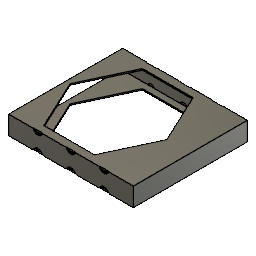
NES Shelf v3 (Autodesk Fusion 360 design; units mm, degrees)
Autodesk Fusion 360 part; units mm, degrees
(part 1 of 2)
sketch "Sketch1" plane through (0, 0, 0) normal (0, 1, 0) x (1, 0, 0)
  line L0 (0, 0) -> (133.9, 0)
  line L1 (133.9, 0) -> (133.9, -119.82)
  line L2 (133.9, -119.82) -> (0, -119.82)
  line L3 (0, -119.82) -> (0, 0)
  line L4 (0, -59.91) -> (109.9, -59.91)
  line L5 (109.9, -59.91) -> (109.9, -6.71)
  line L6 (109.9, -6.71) -> (0, -6.71)
  line L7 (0, -6.71) -> (0, -59.91)
  line L8 (0, -59.91) -> (109.9, -59.91)
  line L9 (109.9, -59.91) -> (109.9, -113.11)
  line L10 (109.9, -113.11) -> (0, -113.11)
  line L11 (0, -113.11) -> (0, -59.91)
  line L12 (109.9, -6.71) -> (109.9, 0)
  line L13 (109.9, -113.11) -> (109.9, -119.82)
  line L14 (109.9, -119.82) -> (109.9, -113.11)
  line L15 (133.9, -113.11) -> (109.9, -113.11)
  line L16 (109.9, -6.71) -> (133.9, -6.71)
  dimension "d1" = 119.82
  dimension "d2" = 133.9
  dimension "d3" = 53.2
  dimension "d4" = 109.9
  dimension "d5" = 53.2
  constraint horizontal L0
  constraint vertical L1
  constraint horizontal L2
  constraint vertical L3
  constraint coincident L0.start L3.end
  constraint horizontal L4
  constraint vertical L5
  constraint horizontal L6
  constraint vertical L7
  constraint midpoint L3 L4.start
  constraint horizontal L8
  constraint vertical L9
  constraint horizontal L10
  constraint vertical L11
  constraint coincident L0 L12.end
  constraint perpendicular L0 L12
  constraint coincident L2 L13.end
  constraint perpendicular L2 L13
  constraint coincident L1 L15.start
  constraint perpendicular L9 L15
  constraint coincident L1 L16.end
  constraint perpendicular L1 L16
  measures "d1" distance of L0.start L2.end
  measures "d2" distance of L0.start L0.end
  measures "d3" distance of L4.start L6.end
  measures "d4" distance of L4.start L4.end
  measures "d5" distance of L4.start L10.end
extrude "Extrude1" add sketch "Sketch1" along normal blind 16.8 contours L0 L3 L6 L12 | L3 L4 L5 L6 L7 L8 | L1 L5 L9 L15 L16 | L3 L4 L8 L9 L10 L11 | L2 L3 L10 L13 L14 makes body 1
sketch "Sketch2" plane through (0, 0, 0) normal (0, 1, 0) x (1, 0, 0)
  line L0 (0, 0) -> (133.9, 0)
  line L1 (133.9, 0) -> (133.9, -119.82)
  line L2 (133.9, -119.82) -> (0, -119.82)
  line L3 (0, -119.82) -> (0, 0)
  line L4 (133.9, 0) -> (135.9, 0)
  line L5 (135.9, 0) -> (135.9, -119.82)
  line L6 (135.9, -119.82) -> (133.9, -119.82)
  line L7 (133.9, -119.82) -> (133.9, 0)
  line L8 (135.9, 0) -> (0, 0)
  line L9 (0, 0) -> (0, 2)
  line L10 (0, 2) -> (135.9, 2)
  line L11 (135.9, 2) -> (135.9, 0)
  line L12 (135.9, -119.82) -> (0, -119.82)
  line L13 (0, -119.82) -> (0, -121.82)
  line L14 (0, -121.82) -> (135.9, -121.82)
  line L15 (135.9, -121.82) -> (135.9, -119.82)
  line L16 (133.9, 0) -> (110.1, 0)
  line L17 (110.1, 0) -> (110.1, -6.5)
  line L18 (110.1, -6.5) -> (133.9, -6.5)
  line L19 (133.9, -6.5) -> (133.9, 0)
  line L20 (133.9, -119.82) -> (110.1, -119.82)
  line L21 (110.1, -119.82) -> (110.1, -113.32)
  line L22 (110.1, -113.32) -> (133.9, -113.32)
  line L23 (133.9, -113.32) -> (133.9, -119.82)
  dimension "d8" = 133.9
  dimension "d9" = 2
  dimension "d10" = 2
  dimension "d11" = 2
  dimension "d12" = 23.8
  dimension "d13" = 6.5
  dimension "d14" = 23.8
  dimension "d15" = 6.5
  constraint horizontal L0
  constraint vertical L1
  constraint horizontal L2
  constraint vertical L3
  constraint coincident L0.start L3.end
  constraint horizontal L4
  constraint vertical L5
  constraint horizontal L6
  constraint vertical L7
  constraint horizontal L8
  constraint vertical L9
  constraint horizontal L10
  constraint vertical L11
  constraint horizontal L12
  constraint vertical L13
  constraint horizontal L14
  constraint vertical L15
  constraint horizontal L16
  constraint vertical L17
  constraint horizontal L18
  constraint vertical L19
  constraint horizontal L20
  constraint vertical L21
  constraint horizontal L22
  constraint vertical L23
  measures "d8" distance of L0.start L0.end
  measures "d9" distance of L0.end L4.end
  measures "d10" distance of L4.end L10.end
  measures "d11" distance of L5.end L14.end
  measures "d12" distance of L0.end L16.end
  measures "d13" distance of L0.end L18.end
  measures "d14" distance of L1.end L20.end
  measures "d15" distance of L1.end L22.end
extrude "Extrude2" add sketch "Sketch2" along normal blind 17 separate body contours L0 L4 L8 L9 L10 L11 L16 | L0 L1 L7 L8 L16 L17 L18 L19 | L2 L6 L12 L13 L14 L15 L20 | L1 L4 L5 L6 L7 L8 L12 L19 L23 | L1 L2 L7 L12 L20 L21 L22 L23 makes body 2
extrude "Extrude3" cut 1 faces at (36.7, 11.3333, 0) along direction (0, 0, -1) blind 0.2 on bodies 2 bodies 2
extrude "Extrude4" cut 1 faces at (73.4, 5.6667, 119.82) along direction (0, 0, 1) blind 0.2 on bodies 2 bodies 2
extrude "Extrude5" add 1 faces at (45.3, 5.6667, -2) along direction (0, 0, -1) blind 0.2 on bodies 2 bodies 2
extrude "Extrude6" add 1 faces at (45.3, 5.6667, 121.82) along direction (0, 0, 1) blind 0.2 on bodies 2 bodies 2
sketch "Sketch3" plane through (0, 0, 0) normal (0, -1, 0) x (1, 0, 0)
  line L0 (110.1, 120.02) -> (110.1, 113.32)
  line L1 (110.1, 113.32) -> (133.9, 113.32)
  line L2 (133.9, 113.32) -> (133.9, 6.5)
  line L3 (133.9, 6.5) -> (110.1, 6.5)
  line L4 (110.1, 6.5) -> (110.1, -0.2)
  line L5 (110.1, -0.2) -> (0, -0.2)
  line L6 (0, -0.2) -> (0, -2.2)
  line L7 (0, -2.2) -> (135.9, -2.2)
  line L8 (135.9, -2.2) -> (135.9, 122.02)
  line L9 (135.9, 122.02) -> (0, 122.02)
  line L10 (0, 122.02) -> (0, 120.02)
  line L11 (0, 120.02) -> (110.1, 120.02)
  line L12 (135.9, -2.2) -> (0, -2.2)
  line L13 (0, -2.2) -> (0, 122.02)
  line L14 (0, 122.02) -> (135.9, 122.02)
  line L15 (135.9, 122.02) -> (135.9, -2.2)
  constraint horizontal L12
  constraint vertical L13
  constraint horizontal L14
  constraint vertical L15
  constraint coincident L9.end L10.start
  constraint coincident L7.end L8.start
extrude "Extrude7" add sketch "Sketch3" along normal blind 1.5 bodies 2
sketch "Sketch4" plane through (0, 17, 0) normal (0, 1, 0) x (-1, 0, 0)
  line L0 (-110.1, 113.32) -> (-110.1, 120.02)
  line L1 (-110.1, 120.02) -> (0, 120.02)
  line L2 (0, 120.02) -> (0, 122.02)
  line L3 (0, 122.02) -> (-135.9, 122.02)
  line L4 (-135.9, 122.02) -> (-135.9, -2.2)
  line L5 (-135.9, -2.2) -> (0, -2.2)
  line L6 (0, -2.2) -> (0, -0.2)
  line L7 (0, -0.2) -> (-110.1, -0.2)
  line L8 (-110.1, -0.2) -> (-110.1, 6.5)
  line L9 (-110.1, 6.5) -> (-133.9, 6.5)
  line L10 (-133.9, 6.5) -> (-133.9, 113.32)
  line L11 (-133.9, 113.32) -> (-110.1, 113.32)
  line L12 (-135.9, -2.2) -> (0, -2.2)
  line L13 (0, -2.2) -> (0, 122.02)
  line L14 (0, 122.02) -> (-135.9, 122.02)
  line L15 (-135.9, 122.02) -> (-135.9, -2.2)
  constraint horizontal L12
  constraint vertical L13
  constraint horizontal L14
  constraint vertical L15
  constraint coincident L2.end L3.start
  constraint coincident L4.end L5.start
extrude "Extrude8" add sketch "Sketch4" along normal blind 1.5 bodies 2
extrude "Extrude9" cut 1 faces at (45.3, 18.5, 39.2067) along direction (0, -1, 0) blind 0.5 on bodies 2 bodies 2
extrude "Extrude10" cut 1 faces at (90.6, -1.5, 39.2067) along direction (0, 1, 0) blind 0.5 on bodies 2 bodies 2
sketch "Sketch5" plane through (0, 0, -2.2) normal (0, 0, -1) x (-1, 0, 0)
  line L0 (-135.9, -1) -> (0, -1)
  line L1 (0, -1) -> (0, 18)
  line L2 (0, 18) -> (-135.9, 18)
  line L3 (-135.9, 18) -> (-135.9, -1)
  line L4 (-67.95, -1) -> (-63.95, -1)
  line L5 (-63.95, -1) -> (-63.95, 0)
  line L6 (-63.95, 0) -> (-67.95, 0)
  line L7 (-67.95, 0) -> (-67.95, -1)
  line L8 (-67.95, 0) -> (-71.95, 0)
  line L9 (-71.95, 0) -> (-71.95, -1)
  line L10 (-71.95, -1) -> (-67.95, -1)
  line L11 (-67.95, -1) -> (-67.95, 0)
  line L12 (-63.95, 0) -> (-71.95, 0)
  line L13 (-71.95, 0) -> (-71.95, 2)
  line L14 (-71.95, 2) -> (-63.95, 2)
  line L15 (-63.95, 2) -> (-63.95, 0)
  dimension "d34" = 4
  dimension "d35" = 1
  dimension "d36" = 1
  dimension "d37" = 4
  dimension "d38" = 8
  dimension "d39" = 2
  constraint horizontal L4
  constraint vertical L5
  constraint horizontal L6
  constraint vertical L7
  constraint midpoint L0 L4.start
  constraint horizontal L8
  constraint vertical L9
  constraint horizontal L10
  constraint vertical L11
  constraint horizontal L12
  constraint vertical L13
  constraint horizontal L14
  constraint vertical L15
  measures "d34" distance of L4.start L4.end
  measures "d35" distance of L4.start L6.end
  measures "d36" distance of L6.end L4.start
  measures "d37" distance of L6.end L8.end
  measures "d38" distance of L5.end L8.end
  measures "d39" distance of L5.end L14.end
extrude "Extrude11" cut sketch "Sketch5" against normal blind 1.5 contours L6 L8 L12 L13 L14 L15 bodies 2
extrude "Extrude12" cut sketch "Sketch5" against normal blind 0.5 contours L0 L7 L8 L9 L10 L11 L12 | L0 L4 L5 L6 L7 L11 L12 bodies 2
sketch "Sketch6" plane through (0, 0, -2.2) normal (0, 0, -1) x (-1, 0, 0)
  line L0 (-71.95, -1) -> (-71.95, 2)
  line L1 (-71.95, 2) -> (-63.95, 2)
  line L2 (-63.95, 2) -> (-63.95, -1)
  line L3 (-63.95, -1) -> (0, -1)
  line L4 (0, -1) -> (0, 18)
  line L5 (0, 18) -> (-135.9, 18)
  line L6 (-135.9, 18) -> (-135.9, -1)
  line L7 (-135.9, -1) -> (-71.95, -1)
  line L8 (-31.975, -1) -> (-27.975, -1)
  line L9 (-27.975, -1) -> (-27.975, 0)
  line L10 (-27.975, 0) -> (-31.975, 0)
  line L11 (-31.975, 0) -> (-31.975, -1)
  line L12 (-31.975, 0) -> (-35.975, 0)
  line L13 (-35.975, 0) -> (-35.975, -1)
  line L14 (-35.975, -1) -> (-31.975, -1)
  line L15 (-31.975, -1) -> (-31.975, 0)
  line L16 (-103.925, -1) -> (-99.925, -1)
  line L17 (-99.925, -1) -> (-99.925, 0)
  line L18 (-99.925, 0) -> (-103.925, 0)
  line L19 (-103.925, 0) -> (-103.925, -1)
  line L20 (-103.925, 0) -> (-107.925, 0)
  line L21 (-107.925, 0) -> (-107.925, -1)
  line L22 (-107.925, -1) -> (-103.925, -1)
  line L23 (-103.925, -1) -> (-103.925, 0)
  line L24 (-107.925, 0) -> (-103.925, 0)
  line L25 (-103.925, 0) -> (-103.925, 2)
  line L26 (-103.925, 2) -> (-107.925, 2)
  line L27 (-107.925, 2) -> (-107.925, 0)
  line L28 (-27.975, 0) -> (-35.975, 0)
  line L29 (-35.975, 0) -> (-35.975, 2)
  line L30 (-35.975, 2) -> (-27.975, 2)
  line L31 (-27.975, 2) -> (-27.975, 0)
  line L32 (-103.925, 2) -> (-99.925, 2)
  line L33 (-99.925, 2) -> (-99.925, 0)
  line L34 (-99.925, 0) -> (-103.925, 0)
  line L35 (-103.925, 0) -> (-103.925, 2)
  dimension "d44" = 4
  dimension "d45" = 1
  dimension "d46" = 4
  dimension "d47" = 4
  dimension "d48" = 4
  dimension "d49" = 4
  dimension "d50" = 8
  constraint horizontal L8
  constraint vertical L9
  constraint horizontal L10
  constraint vertical L11
  constraint midpoint L3 L8.start
  constraint horizontal L12
  constraint vertical L13
  constraint horizontal L14
  constraint vertical L15
  constraint horizontal L16
  constraint vertical L17
  constraint horizontal L18
  constraint vertical L19
  constraint midpoint L7 L16.start
  constraint horizontal L20
  constraint vertical L21
  constraint horizontal L22
  constraint vertical L23
  constraint horizontal L24
  constraint vertical L25
  constraint horizontal L26
  constraint vertical L27
  constraint horizontal L28
  constraint vertical L29
  constraint horizontal L30
  constraint vertical L31
  constraint horizontal L32
  constraint vertical L33
  constraint horizontal L34
  constraint vertical L35
  measures "d44" distance of L8.start L8.end
  measures "d45" distance of L8.start L10.end
  measures "d46" distance of L10.end L12.end
  measures "d47" distance of L16.start L16.end
  measures "d48" distance of L18.end L20.end
  measures "d49" distance of L20.end L18.end
  measures "d50" distance of L9.end L12.end
extrude "Extrude13" cut sketch "Sketch6" against normal blind 1.5 contours L18 L25 L32 L33 L34 L35 | L20 L24 L25 L26 L27 L35 | L10 L12 L28 L29 L30 L31 bodies 2
extrude "Extrude14" cut sketch "Sketch6" against normal blind 0.5 contours L7 L16 L17 L18 L19 L23 L34 | L7 L19 L20 L21 L22 L23 L24 | L3 L11 L12 L13 L14 L15 L28 | L3 L8 L9 L10 L11 L15 L28 bodies 2
sketch "Sketch7" plane through (135.9, 0, 0) normal (1, 0, 0) x (0, 0, -1)
  line L0 (-122.02, -1) -> (2.2, -1)
  line L1 (2.2, -1) -> (2.2, 18)
  line L2 (2.2, 18) -> (-122.02, 18)
  line L3 (-122.02, 18) -> (-122.02, -1)
  line L4 (-59.91, -1) -> (-55.91, -1)
  line L5 (-55.91, -1) -> (-55.91, 0)
  line L6 (-55.91, 0) -> (-59.91, 0)
  line L7 (-59.91, 0) -> (-59.91, -1)
  line L8 (-59.91, 0) -> (-63.91, 0)
  line L9 (-63.91, 0) -> (-63.91, -1)
  line L10 (-63.91, -1) -> (-59.91, -1)
  line L11 (-59.91, -1) -> (-59.91, 0)
  line L12 (-63.91, 0) -> (-55.91, 0)
  line L13 (-55.91, 0) -> (-55.91, 2)
  line L14 (-55.91, 2) -> (-63.91, 2)
  line L15 (-63.91, 2) -> (-63.91, 0)
  dimension "d55" = 4
  dimension "d56" = 4
  dimension "d57" = 1
  dimension "d58" = 8
  dimension "d59" = 2
  constraint horizontal L4
  constraint vertical L5
  constraint horizontal L6
  constraint vertical L7
  constraint midpoint L0 L4.start
  constraint horizontal L8
  constraint vertical L9
  constraint horizontal L10
  constraint vertical L11
  constraint horizontal L12
  constraint vertical L13
  constraint horizontal L14
  constraint vertical L15
  measures "d55" distance of L4.start L4.end
  measures "d56" distance of L6.end L8.end
  measures "d57" distance of L6.end L4.start
  measures "d58" distance of L8.end L5.end
  measures "d59" distance of L8.end L14.end
extrude "Extrude15" cut sketch "Sketch7" against normal blind 1.5 contours L6 L8 L12 L13 L14 L15 bodies 2
extrude "Extrude16" cut sketch "Sketch7" against normal blind 0.5 contours L0 L7 L8 L9 L10 L11 L12 | L0 L4 L5 L6 L7 L11 L12 bodies 2
sketch "Sketch8" plane through (135.9, 0, 0) normal (1, 0, 0) x (0, 0, -1)
  line L0 (-55.91, 2) -> (-55.91, -1)
  line L1 (-55.91, -1) -> (2.2, -1)
  line L2 (2.2, -1) -> (2.2, 18)
  line L3 (2.2, 18) -> (-122.02, 18)
  line L4 (-122.02, 18) -> (-122.02, -1)
  line L5 (-122.02, -1) -> (-63.91, -1)
  line L6 (-63.91, -1) -> (-63.91, 2)
  line L7 (-63.91, 2) -> (-55.91, 2)
  line L8 (-26.855, -1) -> (-22.855, -1)
  line L9 (-22.855, -1) -> (-22.855, 0)
  line L10 (-22.855, 0) -> (-26.855, 0)
  line L11 (-26.855, 0) -> (-26.855, -1)
  line L12 (-26.855, 0) -> (-30.855, 0)
  line L13 (-30.855, 0) -> (-30.855, -1)
  line L14 (-30.855, -1) -> (-26.855, -1)
  line L15 (-26.855, -1) -> (-26.855, 0)
  line L16 (-30.855, 0) -> (-22.855, 0)
  line L17 (-22.855, 0) -> (-22.855, 2)
  line L18 (-22.855, 2) -> (-30.855, 2)
  line L19 (-30.855, 2) -> (-30.855, 0)
  line L20 (-92.965, -1) -> (-96.965, -1)
  line L21 (-96.965, -1) -> (-96.965, 0)
  line L22 (-96.965, 0) -> (-92.965, 0)
  line L23 (-92.965, 0) -> (-92.965, -1)
  line L24 (-92.965, 0) -> (-88.965, 0)
  line L25 (-88.965, 0) -> (-88.965, -1)
  line L26 (-88.965, -1) -> (-92.965, -1)
  line L27 (-92.965, -1) -> (-92.965, 0)
  line L28 (-88.965, 0) -> (-96.965, 0)
  line L29 (-96.965, 0) -> (-96.965, 2)
  line L30 (-96.965, 2) -> (-88.965, 2)
  line L31 (-88.965, 2) -> (-88.965, 0)
  dimension "d64" = 4
  dimension "d65" = 4
  dimension "d66" = 8
  dimension "d67" = 2
  dimension "d68" = 4
  dimension "d69" = 4
  dimension "d70" = 1
  dimension "d71" = 8
  dimension "d72" = 2
  constraint horizontal L8
  constraint vertical L9
  constraint horizontal L10
  constraint vertical L11
  constraint midpoint L1 L8.start
  constraint horizontal L12
  constraint vertical L13
  constraint horizontal L14
  constraint vertical L15
  constraint horizontal L16
  constraint vertical L17
  constraint horizontal L18
  constraint vertical L19
  constraint horizontal L20
  constraint vertical L21
  constraint horizontal L22
  constraint vertical L23
  constraint midpoint L5 L20.start
  constraint horizontal L24
  constraint vertical L25
  constraint horizontal L26
  constraint vertical L27
  constraint horizontal L28
  constraint vertical L29
  constraint horizontal L30
  constraint vertical L31
  measures "d64" distance of L8.start L8.end
  measures "d65" distance of L10.end L12.end
  measures "d66" distance of L12.end L9.end
  measures "d67" distance of L12.end L18.end
  measures "d68" distance of L20.start L20.end
  measures "d69" distance of L22.end L24.end
  measures "d70" distance of L22.end L20.start
  measures "d71" distance of L24.end L21.end
  measures "d72" distance of L24.end L30.end
extrude "Extrude17" cut sketch "Sketch8" against normal blind 1.5 contours L10 L12 L16 L17 L18 L19 | L22 L24 L28 L29 L30 L31 bodies 2
extrude "Extrude18" cut sketch "Sketch8" against normal blind 0.5 contours L1 L11 L12 L13 L14 L15 L16 | L1 L8 L9 L10 L11 L15 L16 | L5 L23 L24 L25 L26 L27 L28 | L5 L20 L21 L22 L23 L27 L28 bodies 2
sketch "Sketch9" plane through (0, 0, 122.02) normal (0, 0, 1) x (1, 0, 0)
  line L0 (0, -1) -> (135.9, -1)
  line L1 (135.9, -1) -> (135.9, 18)
  line L2 (135.9, 18) -> (0, 18)
  line L3 (0, 18) -> (0, -1)
  line L4 (67.95, -1) -> (63.95, -1)
  line L5 (63.95, -1) -> (63.95, 0)
  line L6 (63.95, 0) -> (67.95, 0)
  line L7 (67.95, 0) -> (67.95, -1)
  line L8 (67.95, 0) -> (71.95, 0)
  line L9 (71.95, 0) -> (71.95, -1)
  line L10 (71.95, -1) -> (67.95, -1)
  line L11 (67.95, -1) -> (67.95, 0)
  line L12 (71.95, 0) -> (63.95, 0)
  line L13 (63.95, 0) -> (63.95, 2)
  line L14 (63.95, 2) -> (71.95, 2)
  line L15 (71.95, 2) -> (71.95, 0)
  dimension "d77" = 1
  dimension "d78" = 4
  dimension "d79" = 1
  dimension "d80" = 4
  dimension "d81" = 2
  constraint horizontal L4
  constraint vertical L5
  constraint horizontal L6
  constraint vertical L7
  constraint midpoint L0 L4.start
  constraint horizontal L8
  constraint vertical L9
  constraint horizontal L10
  constraint vertical L11
  constraint horizontal L12
  constraint vertical L13
  constraint horizontal L14
  constraint vertical L15
  measures "d77" distance of L4.start L6.end
  measures "d78" distance of L4.start L4.end
  measures "d79" distance of L6.end L4.start
  measures "d80" distance of L6.end L8.end
  measures "d81" distance of L8.end L14.end
extrude "Extrude19" cut sketch "Sketch9" against normal blind 1.5 contours L6 L8 L12 L13 L14 L15 bodies 2
extrude "Extrude20" cut sketch "Sketch9" against normal blind 0.5 contours L0 L4 L5 L6 L7 L11 L12 | L0 L7 L8 L9 L10 L11 L12 bodies 2
sketch "Sketch10" plane through (0, 0, 122.02) normal (0, 0, 1) x (1, 0, 0)
  line L0 (71.95, 2) -> (71.95, -1)
  line L1 (71.95, -1) -> (135.9, -1)
  line L2 (135.9, -1) -> (135.9, 18)
  line L3 (135.9, 18) -> (0, 18)
  line L4 (0, 18) -> (0, -1)
  line L5 (0, -1) -> (63.95, -1)
  line L6 (63.95, -1) -> (63.95, 2)
  line L7 (63.95, 2) -> (71.95, 2)
  line L8 (31.975, -1) -> (35.975, -1)
  line L9 (35.975, -1) -> (35.975, 0)
  line L10 (35.975, 0) -> (31.975, 0)
  line L11 (31.975, 0) -> (31.975, -1)
  line L12 (31.975, 0) -> (27.975, 0)
  line L13 (27.975, 0) -> (27.975, -1)
  line L14 (27.975, -1) -> (31.975, -1)
  line L15 (31.975, -1) -> (31.975, 0)
  line L16 (27.975, 0) -> (35.975, 0)
  line L17 (35.975, 0) -> (35.975, 2)
  line L18 (35.975, 2) -> (27.975, 2)
  line L19 (27.975, 2) -> (27.975, 0)
  line L20 (103.925, -1) -> (107.925, -1)
  line L21 (107.925, -1) -> (107.925, 0)
  line L22 (107.925, 0) -> (103.925, 0)
  line L23 (103.925, 0) -> (103.925, -1)
  line L24 (103.925, 0) -> (99.925, 0)
  line L25 (99.925, 0) -> (99.925, -1)
  line L26 (99.925, -1) -> (103.925, -1)
  line L27 (103.925, -1) -> (103.925, 0)
  line L28 (99.925, 0) -> (107.925, 0)
  line L29 (107.925, 0) -> (107.925, 2)
  line L30 (107.925, 2) -> (99.925, 2)
  line L31 (99.925, 2) -> (99.925, 0)
  dimension "d86" = 4
  dimension "d87" = 4
  dimension "d88" = 1
  dimension "d89" = 8
  dimension "d90" = 2
  dimension "d91" = 4
  dimension "d92" = 4
  dimension "d93" = 8
  constraint horizontal L8
  constraint vertical L9
  constraint horizontal L10
  constraint vertical L11
  constraint midpoint L5 L8.start
  constraint horizontal L12
  constraint vertical L13
  constraint horizontal L14
  constraint vertical L15
  constraint horizontal L16
  constraint vertical L17
  constraint horizontal L18
  constraint vertical L19
  constraint horizontal L20
  constraint vertical L21
  constraint horizontal L22
  constraint vertical L23
  constraint midpoint L1 L20.start
  constraint horizontal L24
  constraint vertical L25
  constraint horizontal L26
  constraint vertical L27
  constraint horizontal L28
  constraint vertical L29
  constraint horizontal L30
  constraint vertical L31
  measures "d86" distance of L8.start L8.end
  measures "d87" distance of L10.end L12.end
  measures "d88" distance of L10.end L8.start
  measures "d89" distance of L12.end L9.end
  measures "d90" distance of L12.end L18.end
  measures "d91" distance of L20.start L20.end
  measures "d92" distance of L22.end L24.end
  measures "d93" distance of L24.end L21.end
extrude "Extrude21" cut sketch "Sketch10" against normal blind 1.5 contours L22 L24 L28 L29 L30 L31 | L10 L12 L16 L17 L18 L19 bodies 2
extrude "Extrude22" cut sketch "Sketch10" against normal blind 0.5 contours L1 L23 L24 L25 L26 L27 L28 | L1 L20 L21 L22 L23 L27 L28 | L5 L8 L9 L10 L11 L15 L16 | L5 L11 L12 L13 L14 L15 L16 bodies 2
sketch "Sketch11" plane through (0, 0, 122.02) normal (0, 0, 1) x (1, 0, 0)
  line L0 (35.975, 2) -> (35.975, -1)
  line L1 (35.975, -1) -> (63.95, -1)
  line L2 (63.95, -1) -> (63.95, 2)
  line L3 (63.95, 2) -> (71.95, 2)
  line L4 (71.95, 2) -> (71.95, -1)
  line L5 (71.95, -1) -> (99.925, -1)
  line L6 (99.925, -1) -> (99.925, 2)
  line L7 (99.925, 2) -> (107.925, 2)
  line L8 (107.925, 2) -> (107.925, -1)
  line L9 (107.925, -1) -> (135.9, -1)
  line L10 (135.9, -1) -> (135.9, 18)
  line L11 (135.9, 18) -> (0, 18)
  line L12 (0, 18) -> (0, -1)
  line L13 (0, -1) -> (27.975, -1)
  line L14 (27.975, -1) -> (27.975, 2)
  line L15 (27.975, 2) -> (35.975, 2)
  line L16 (27.975, 2) -> (35.975, 2)
  line L17 (35.975, 2) -> (35.975, 18)
  line L18 (35.975, 18) -> (27.975, 18)
  line L19 (27.975, 18) -> (27.975, 2)
  line L20 (63.95, 2) -> (71.95, 2)
  line L21 (71.95, 2) -> (71.95, 18)
  line L22 (71.95, 18) -> (63.95, 18)
  line L23 (63.95, 18) -> (63.95, 2)
  line L24 (99.925, 2) -> (107.925, 2)
  line L25 (107.925, 2) -> (107.925, 18)
  line L26 (107.925, 18) -> (99.925, 18)
  line L27 (99.925, 18) -> (99.925, 2)
  line L28 (107.925, 18) -> (107.925, 17)
  line L29 (107.925, 18) -> (107.925, 17)
  line L30 (107.925, 17) -> (27.975, 17)
  line L31 (107.925, 17) -> (107.925, 15)
  line L32 (107.925, 17) -> (107.925, 15)
  line L33 (107.925, 15) -> (27.975, 15)
  dimension "d98" = 8
  dimension "d99" = 8
  dimension "d100" = 8
  dimension "d101" = 1
  constraint horizontal L16
  constraint vertical L17
  constraint horizontal L18
  constraint vertical L19
  constraint coincident L14.end L15.start
  constraint horizontal L20
  constraint vertical L21
  constraint horizontal L22
  constraint vertical L23
  constraint coincident L2.end L3.start
  constraint horizontal L24
  constraint vertical L25
  constraint horizontal L26
  constraint vertical L27
  constraint coincident L6.end L7.start
  constraint coincident L25 L28.end
  constraint perpendicular L26 L28
  constraint coincident L19 L30.end
  constraint coincident L25 L31.end
  constraint parallel L25 L31
  constraint parallel L31 L32
  constraint coincident L19 L33.end
  constraint perpendicular L19 L33
  measures "d98" distance of L14.end L0.start
  measures "d99" distance of L2.end L3.end
  measures "d100" distance of L6.end L7.end
  measures "d101" distance of L25.end L28.end
extrude "Extrude23" cut sketch "Sketch11" against normal blind 1.5 contours L17 L19 L30 L33 | L21 L23 L30 L33 | L25 L27 L30 L31 L32 L33 bodies 2
extrude "Extrude24" cut sketch "Sketch11" against normal blind 0.5 contours L11 L17 L18 L19 L30 | L11 L21 L22 L23 L30 | L11 L25 L26 L27 L28 L29 L30 bodies 2
sketch "Sketch12" plane through (135.9, 0, 0) normal (1, 0, 0) x (0, 0, -1)
  line L0 (-96.965, -1) -> (-96.965, 2)
  line L1 (-96.965, 2) -> (-88.965, 2)
  line L2 (-88.965, 2) -> (-88.965, -1)
  line L3 (-88.965, -1) -> (-63.91, -1)
  line L4 (-63.91, -1) -> (-63.91, 2)
  line L5 (-63.91, 2) -> (-55.91, 2)
  line L6 (-55.91, 2) -> (-55.91, -1)
  line L7 (-55.91, -1) -> (-30.855, -1)
  line L8 (-30.855, -1) -> (-30.855, 2)
  line L9 (-30.855, 2) -> (-22.855, 2)
  line L10 (-22.855, 2) -> (-22.855, -1)
  line L11 (-22.855, -1) -> (2.2, -1)
  line L12 (2.2, -1) -> (2.2, 18)
  line L13 (2.2, 18) -> (-122.02, 18)
  line L14 (-122.02, 18) -> (-122.02, -1)
  line L15 (-122.02, -1) -> (-96.965, -1)
  line L16 (-96.965, -1) -> (-88.965, -1)
  line L17 (-88.965, -1) -> (-88.965, 17)
  line L18 (-88.965, 17) -> (-96.965, 17)
  line L19 (-96.965, 17) -> (-96.965, -1)
  line L20 (-63.91, -1) -> (-55.91, -1)
  line L21 (-55.91, -1) -> (-55.91, 17)
  line L22 (-55.91, 17) -> (-63.91, 17)
  line L23 (-63.91, 17) -> (-63.91, -1)
  line L24 (-30.855, -1) -> (-22.855, -1)
  line L25 (-22.855, -1) -> (-22.855, 17)
  line L26 (-22.855, 17) -> (-30.855, 17)
  line L27 (-30.855, 17) -> (-30.855, -1)
  line L28 (-22.855, 17) -> (-30.855, 17)
  line L29 (-30.855, 17) -> (-30.855, 15)
  line L30 (-30.855, 15) -> (-22.855, 15)
  line L31 (-22.855, 15) -> (-22.855, 17)
  line L32 (-55.91, 17) -> (-63.91, 17)
  line L33 (-63.91, 17) -> (-63.91, 15)
  line L34 (-63.91, 15) -> (-55.91, 15)
  line L35 (-55.91, 15) -> (-55.91, 17)
  line L36 (-96.965, 17) -> (-88.965, 17)
  line L37 (-88.965, 17) -> (-88.965, 15)
  line L38 (-88.965, 15) -> (-96.965, 15)
  line L39 (-96.965, 15) -> (-96.965, 17)
  dimension "d106" = 18
  dimension "d107" = 8
  dimension "d108" = 18
  dimension "d109" = 8
  dimension "d110" = 18
  dimension "d111" = 8
  dimension "d112" = 2
  dimension "d113" = 2
  dimension "d114" = 2
  constraint horizontal L16
  constraint vertical L17
  constraint horizontal L18
  constraint vertical L19
  constraint coincident L0.start L15.end
  constraint horizontal L20
  constraint vertical L21
  constraint horizontal L22
  constraint vertical L23
  constraint coincident L3.end L4.start
  constraint horizontal L24
  constraint vertical L25
  constraint horizontal L26
  constraint vertical L27
  constraint coincident L7.end L8.start
  constraint horizontal L28
  constraint vertical L29
  constraint horizontal L30
  constraint vertical L31
  constraint horizontal L32
  constraint vertical L33
  constraint horizontal L34
  constraint vertical L35
  constraint horizontal L36
  constraint vertical L37
  constraint horizontal L38
  constraint vertical L39
  measures "d106" distance of L0.start L18.end
  measures "d107" distance of L0.start L2.end
  measures "d108" distance of L3.end L22.end
  measures "d109" distance of L3.end L6.end
  measures "d110" distance of L7.end L26.end
  measures "d111" distance of L7.end L10.end
  measures "d112" distance of L25.end L30.end
  measures "d113" distance of L21.end L34.end
  measures "d114" distance of L18.end L38.end
extrude "Extrude25" cut sketch "Sketch12" against normal blind 1.5 contours L17 L18 L19 L36 L37 L38 L39 | L21 L22 L23 L32 L33 L34 L35 | L25 L26 L27 L28 L29 L30 L31 bodies 2
sketch "Sketch13" plane through (135.9, 0, 0) normal (1, 0, 0) x (0, 0, -1)
  line L0 (-88.965, 17) -> (-88.965, 15)
  line L1 (-88.965, 15) -> (-96.965, 15)
  line L2 (-96.965, 15) -> (-96.965, 17)
  line L3 (-96.965, 17) -> (-88.965, 17)
  line L4 (-63.91, 17) -> (-55.91, 17)
  line L5 (-55.91, 17) -> (-55.91, 15)
  line L6 (-55.91, 15) -> (-63.91, 15)
  line L7 (-63.91, 15) -> (-63.91, 17)
  line L8 (-30.855, 17) -> (-22.855, 17)
  line L9 (-22.855, 17) -> (-22.855, 15)
  line L10 (-22.855, 15) -> (-30.855, 15)
  line L11 (-30.855, 15) -> (-30.855, 17)
  line L12 (-96.965, -1) -> (-96.965, 2)
  line L13 (-96.965, 2) -> (-88.965, 2)
  line L14 (-88.965, 2) -> (-88.965, -1)
  line L15 (-88.965, -1) -> (-63.91, -1)
  line L16 (-63.91, -1) -> (-63.91, 2)
  line L17 (-63.91, 2) -> (-55.91, 2)
  line L18 (-55.91, 2) -> (-55.91, -1)
  line L19 (-55.91, -1) -> (-30.855, -1)
  line L20 (-30.855, -1) -> (-30.855, 2)
  line L21 (-30.855, 2) -> (-22.855, 2)
  line L22 (-22.855, 2) -> (-22.855, -1)
  line L23 (-22.855, -1) -> (2.2, -1)
  line L24 (2.2, -1) -> (2.2, 18)
  line L25 (2.2, 18) -> (-122.02, 18)
  line L26 (-122.02, 18) -> (-122.02, -1)
  line L27 (-122.02, -1) -> (-96.965, -1)
  line L28 (-22.855, 17) -> (-30.855, 17)
  line L29 (-30.855, 17) -> (-30.855, 18)
  line L30 (-30.855, 18) -> (-22.855, 18)
  line L31 (-22.855, 18) -> (-22.855, 17)
  line L32 (-55.91, 17) -> (-63.91, 17)
  line L33 (-63.91, 17) -> (-63.91, 18)
  line L34 (-63.91, 18) -> (-55.91, 18)
  line L35 (-55.91, 18) -> (-55.91, 17)
  line L36 (-96.965, 17) -> (-88.965, 17)
  line L37 (-88.965, 17) -> (-88.965, 18)
  line L38 (-88.965, 18) -> (-96.965, 18)
  line L39 (-96.965, 18) -> (-96.965, 17)
  dimension "d117" = 8
  dimension "d118" = 8
  dimension "d119" = 1
  dimension "d120" = 8
  constraint horizontal L28
  constraint vertical L29
  constraint horizontal L30
  constraint vertical L31
  constraint coincident L8.end L9.start
  constraint horizontal L32
  constraint vertical L33
  constraint horizontal L34
  constraint vertical L35
  constraint coincident L4.end L5.start
  constraint horizontal L36
  constraint vertical L37
  constraint horizontal L38
  constraint vertical L39
  constraint coincident L2.end L3.start
  measures "d117" distance of L8.end L8.start
  measures "d118" distance of L4.end L4.start
  measures "d119" distance of L4.end L34.end
  measures "d120" distance of L2.end L0.start
extrude "Extrude26" cut sketch "Sketch13" against normal blind 0.5 contours L3 L25 L36 L37 L38 L39 | L4 L25 L32 L33 L34 L35 | L8 L25 L28 L29 L30 L31 bodies 2
sketch "Sketch14" plane through (0, 0, -2.2) normal (0, 0, -1) x (-1, 0, 0)
  line L0 (-99.925, 2) -> (-99.925, -1)
  line L1 (-99.925, -1) -> (-71.95, -1)
  line L2 (-71.95, -1) -> (-71.95, 2)
  line L3 (-71.95, 2) -> (-63.95, 2)
  line L4 (-63.95, 2) -> (-63.95, -1)
  line L5 (-63.95, -1) -> (-35.975, -1)
  line L6 (-35.975, -1) -> (-35.975, 2)
  line L7 (-35.975, 2) -> (-27.975, 2)
  line L8 (-27.975, 2) -> (-27.975, -1)
  line L9 (-27.975, -1) -> (0, -1)
  line L10 (0, -1) -> (0, 18)
  line L11 (0, 18) -> (-135.9, 18)
  line L12 (-135.9, 18) -> (-135.9, -1)
  line L13 (-135.9, -1) -> (-107.925, -1)
  line L14 (-107.925, -1) -> (-107.925, 2)
  line L15 (-107.925, 2) -> (-99.925, 2)
  line L16 (-107.925, 2) -> (-99.925, 2)
  line L17 (-99.925, 2) -> (-99.925, 17)
  line L18 (-99.925, 17) -> (-107.925, 17)
  line L19 (-107.925, 17) -> (-107.925, 2)
  line L20 (-71.95, 2) -> (-63.95, 2)
  line L21 (-63.95, 2) -> (-63.95, 17)
  line L22 (-63.95, 17) -> (-71.95, 17)
  line L23 (-71.95, 17) -> (-71.95, 2)
  line L24 (-35.975, 2) -> (-27.975, 2)
  line L25 (-27.975, 2) -> (-27.975, 17)
  line L26 (-27.975, 17) -> (-35.975, 17)
  line L27 (-35.975, 17) -> (-35.975, 2)
  line L28 (-27.975, 17) -> (-35.975, 17)
  line L29 (-35.975, 17) -> (-35.975, 15)
  line L30 (-35.975, 15) -> (-27.975, 15)
  line L31 (-27.975, 15) -> (-27.975, 17)
  line L32 (-63.95, 17) -> (-72, 17)
  line L33 (-72, 17) -> (-72, 15)
  line L34 (-72, 15) -> (-63.95, 15)
  line L35 (-63.95, 15) -> (-63.95, 17)
  line L36 (-99.925, 17) -> (-107.925, 17)
  line L37 (-107.925, 17) -> (-107.925, 15)
  line L38 (-107.925, 15) -> (-99.925, 15)
  line L39 (-99.925, 15) -> (-99.925, 17)
  dimension "d123" = 15
  dimension "d124" = 15
  dimension "d125" = 8
  dimension "d126" = 15
  dimension "d127" = 8
  dimension "d128" = 2
  dimension "d129" = 2
  dimension "d130" = 2
  constraint horizontal L16
  constraint vertical L17
  constraint horizontal L18
  constraint vertical L19
  constraint coincident L14.end L15.start
  constraint horizontal L20
  constraint vertical L21
  constraint horizontal L22
  constraint vertical L23
  constraint coincident L2.end L3.start
  constraint horizontal L24
  constraint vertical L25
  constraint horizontal L26
  constraint vertical L27
  constraint coincident L6.end L7.start
  constraint horizontal L28
  constraint vertical L29
  constraint horizontal L30
  constraint vertical L31
  constraint horizontal L32
  constraint vertical L33
  constraint horizontal L34
  constraint vertical L35
  constraint horizontal L36
  constraint vertical L37
  constraint horizontal L38
  constraint vertical L39
  measures "d123" distance of L14.end L18.end
  measures "d124" distance of L2.end L22.end
  measures "d125" distance of L2.end L3.end
  measures "d126" distance of L6.end L26.end
  measures "d127" distance of L6.end L7.end
  measures "d128" distance of L25.end L30.end
  measures "d129" distance of L21.end L34.end
  measures "d130" distance of L17.end L38.end
extrude "Extrude27" cut sketch "Sketch14" against normal blind 1.5 contours L17 L18 L19 L36 L37 L38 L39 | L21 L22 L23 L32 L34 L35 | L25 L26 L27 L28 L29 L30 L31 bodies 2
sketch "Sketch15" plane through (0, 0, -2.2) normal (0, 0, -1) x (-1, 0, 0)
  line L0 (-107.925, 17) -> (-99.925, 17)
  line L1 (-99.925, 17) -> (-99.925, 15)
  line L2 (-99.925, 15) -> (-107.925, 15)
  line L3 (-107.925, 15) -> (-107.925, 17)
  line L4 (-71.95, 17) -> (-63.95, 17)
  line L5 (-63.95, 17) -> (-63.95, 15)
  line L6 (-63.95, 15) -> (-71.95, 15)
  line L7 (-71.95, 15) -> (-71.95, 17)
  line L8 (-35.975, 17) -> (-27.975, 17)
  line L9 (-27.975, 17) -> (-27.975, 15)
  line L10 (-27.975, 15) -> (-35.975, 15)
  line L11 (-35.975, 15) -> (-35.975, 17)
  line L12 (-99.925, 2) -> (-99.925, -1)
  line L13 (-99.925, -1) -> (-71.95, -1)
  line L14 (-71.95, -1) -> (-71.95, 2)
  line L15 (-71.95, 2) -> (-63.95, 2)
  line L16 (-63.95, 2) -> (-63.95, -1)
  line L17 (-63.95, -1) -> (-35.975, -1)
  line L18 (-35.975, -1) -> (-35.975, 2)
  line L19 (-35.975, 2) -> (-27.975, 2)
  line L20 (-27.975, 2) -> (-27.975, -1)
  line L21 (-27.975, -1) -> (0, -1)
  line L22 (0, -1) -> (0, 18)
  line L23 (0, 18) -> (-135.9, 18)
  line L24 (-135.9, 18) -> (-135.9, -1)
  line L25 (-135.9, -1) -> (-107.925, -1)
  line L26 (-107.925, -1) -> (-107.925, 2)
  line L27 (-107.925, 2) -> (-99.925, 2)
  line L28 (-107.925, 17) -> (-99.925, 17)
  line L29 (-99.925, 17) -> (-99.925, 18)
  line L30 (-99.925, 18) -> (-107.925, 18)
  line L31 (-107.925, 18) -> (-107.925, 17)
  line L32 (-71.95, 18) -> (-63.95, 18)
  line L33 (-63.95, 18) -> (-63.95, 17)
  line L34 (-63.95, 17) -> (-71.95, 17)
  line L35 (-71.95, 17) -> (-71.95, 18)
  line L36 (-35.975, 18) -> (-27.975, 18)
  line L37 (-27.975, 18) -> (-27.975, 17)
  line L38 (-27.975, 17) -> (-35.975, 17)
  line L39 (-35.975, 17) -> (-35.975, 18)
  point P0 (-99.925, 18)
  point P1 (-71.95, 18)
  point P2 (-35.975, 18)
  constraint horizontal L28
  constraint vertical L29
  constraint horizontal L30
  constraint vertical L31
  constraint coincident P0 L29.end
  constraint coincident L0.start L3.end
  constraint horizontal L32
  constraint vertical L33
  constraint horizontal L34
  constraint vertical L35
  constraint coincident L4.end L5.start
  constraint coincident P1 L32.start
  constraint horizontal L36
  constraint vertical L37
  constraint horizontal L38
  constraint vertical L39
  constraint coincident L8.end L9.start
  constraint coincident P2 L36.start
extrude "Extrude28" cut sketch "Sketch15" against normal blind 0.5 contours L0 L23 L28 L29 L30 L31 | L4 L23 L32 L33 L34 L35 | L8 L23 L36 L37 L38 L39 bodies 2
extrude "Extrude29" cut 1 faces at (107.925, 15.6667, -1.5333) along direction (1, 0, 0) blind 1 on bodies 2 bodies 2
extrude "Extrude30" cut 1 faces at (99.925, 15.6667, -1.5333) along direction (-1, 0, 0) blind 1 on bodies 2 bodies 2
extrude "Extrude31" cut 1 faces at (107.925, 1.3333, -1.5333) along direction (1, 0, 0) blind 1 on bodies 2 bodies 2
extrude "Extrude32" cut 1 faces at (99.925, 1.3333, -1.5333) along direction (-1, 0, 0) blind 1 on bodies 2 bodies 2
extrude "Extrude33" cut 1 faces at (63.95, 1.3333, -1.5333) along direction (-1, 0, 0) blind 1 on bodies 2 bodies 2
extrude "Extrude34" cut 1 faces at (27.975, 15.6667, -1.5333) along direction (-1, 0, 0) blind 1 on bodies 2 bodies 2
extrude "Extrude35" cut 2 faces at (71.95, 15.6667, -1.5333) (71.95, 1.3333, -1.5333) along direction (1, 0, 0) blind 1 on bodies 2 bodies 2
extrude "Extrude36" cut 2 faces at (35.975, 15.6667, -1.5333) (35.975, 1.3333, -1.5333) along direction (1, 0, 0) blind 1 on bodies 2 bodies 2
chamfer "Chamfer1" distance 3 angle 45 1 edges at (26.975, 15, -1.45) on bodies 2
chamfer "Chamfer2" distance 3 angle 45 1 edges at (63.95, 15, -1.45) on bodies 2
chamfer "Chamfer3" distance 3 angle 45 1 edges at (98.925, 15, -1.45) on bodies 2
chamfer "Chamfer4" distance 3 angle 45 1 edges at (108.925, 15, -1.45) on bodies 2
chamfer "Chamfer5" distance 3 angle 45 1 edges at (72.95, 15, -1.45) on bodies 2
chamfer "Chamfer6" distance 3 angle 45 1 edges at (36.975, 15, -1.45) on bodies 2
chamfer "Chamfer7" distance 3 angle 45 1 edges at (27.975, 2, -1.45) on bodies 2
chamfer "Chamfer8" distance 3 angle 45 1 edges at (62.95, 2, -1.45) on bodies 2
chamfer "Chamfer9" distance 3 angle 45 1 edges at (98.925, 2, -1.45) on bodies 2
chamfer "Chamfer10" distance 3 angle 45 1 edges at (108.925, 2, -1.45) on bodies 2
chamfer "Chamfer11" distance 3 angle 45 1 edges at (72.95, 2, -1.45) on bodies 2
chamfer "Chamfer12" distance 3 angle 45 1 edges at (36.975, 2, -1.45) on bodies 2
extrude "Extrude37" cut 1 faces at (107.925, 15.6667, 121.3533) along direction (1, 0, 0) blind 1 on bodies 2 bodies 2
extrude "Extrude38" cut 1 faces at (71.95, 15.6667, 121.3533) along direction (1, 0, 0) blind 1 on bodies 2 bodies 2
extrude "Extrude39" cut 1 faces at (35.975, 15.6667, 121.3533) along direction (1, 0, 0) blind 1 on bodies 2 bodies 2
chamfer "Chamfer13" distance 3 angle 45 1 edges at (36.975, 15, 121.27) on bodies 2
chamfer "Chamfer14" distance 3 angle 45 1 edges at (72.95, 15, 121.27) on bodies 2
chamfer "Chamfer15" distance 3 angle 45 1 edges at (108.925, 15, 121.27) on bodies 2
extrude "Extrude40" cut 1 faces at (99.925, 15.6667, 121.3533) along direction (-1, 0, 0) blind 1 on bodies 2 bodies 2
chamfer "Chamfer16" distance 3 angle 45 1 edges at (98.925, 15, 121.27) on bodies 2
extrude "Extrude41" cut 1 faces at (63.95, 15.6667, 121.3533) along direction (-1, 0, 0) blind 1 on bodies 2 bodies 2
chamfer "Chamfer17" distance 3 angle 45 1 edges at (62.95, 15, 121.27) on bodies 2
extrude "Extrude42" cut 1 faces at (27.975, 15.6667, 121.3533) along direction (-1, 0, 0) blind 1 on bodies 2 bodies 2
chamfer "Chamfer18" distance 3 angle 45 1 edges at (26.975, 15, 121.27) on bodies 2
extrude "Extrude43" cut 1 faces at (35.975, 1.3333, 121.3533) along direction (1, 0, 0) blind 1 on bodies 2 bodies 2
chamfer "Chamfer19" distance 3 angle 45 1 edges at (36.975, 2, 121.27) on bodies 2
extrude "Extrude44" cut 1 faces at (71.95, 1.3333, 121.3533) along direction (1, 0, 0) blind 1 on bodies 2 bodies 2
chamfer "Chamfer20" distance 3 angle 45 1 edges at (72.95, 2, 121.27) on bodies 2
extrude "Extrude45" cut 1 faces at (107.925, 1.3333, 121.3533) along direction (1, 0, 0) blind 1 on bodies 2 bodies 2
chamfer "Chamfer21" distance 3 angle 45 1 edges at (108.925, 2, 121.27) on bodies 2
extrude "Extrude46" cut 1 faces at (99.925, 1.3333, 121.3533) along direction (-1, 0, 0) blind 1 on bodies 2 bodies 2
chamfer "Chamfer22" distance 3 angle 45 1 edges at (98.925, 2, 121.27) on bodies 2
extrude "Extrude47" cut 1 faces at (63.95, 1.3333, 121.3533) along direction (-1, 0, 0) blind 1 on bodies 2 bodies 2
chamfer "Chamfer23" distance 3 angle 45 1 edges at (62.95, 2, 121.27) on bodies 2
extrude "Extrude48" cut 1 faces at (27.975, 1.3333, 121.3533) along direction (-1, 0, 0) blind 1 on bodies 2 bodies 2
chamfer "Chamfer24" distance 3 angle 45 1 edges at (26.975, 2, 121.27) on bodies 2
extrude "Extrude49" cut 1 faces at (135.2333, 1.3333, 96.965) along direction (0, 0, 1) blind 1 on bodies 2 bodies 2
chamfer "Chamfer25" distance 3 angle 45 1 edges at (135.15, 2, 97.965) on bodies 2
extrude "Extrude50" cut 1 faces at (135.2333, 1.3333, 63.91) along direction (0, 0, 1) blind 1 on bodies 2 bodies 2
chamfer "Chamfer26" distance 3 angle 45 1 edges at (135.15, 2, 64.91) on bodies 2
extrude "Extrude51" cut 1 faces at (135.2333, 1.3333, 30.855) along direction (0, 0, 1) blind 1 on bodies 2 bodies 2
chamfer "Chamfer27" distance 3 angle 45 1 edges at (135.15, 2, 31.855) on bodies 2
extrude "Extrude52" cut 1 faces at (135.2333, 1.3333, 22.855) along direction (0, 0, -1) blind 1 on bodies 2 bodies 2
chamfer "Chamfer28" distance 3 angle 45 1 edges at (135.15, 2, 21.855) on bodies 2
extrude "Extrude53" cut 1 faces at (135.2333, 1.3333, 55.91) along direction (0, 0, -1) blind 1 on bodies 2 bodies 2
chamfer "Chamfer29" distance 3 angle 45 1 edges at (135.15, 2, 54.91) on bodies 2
extrude "Extrude54" cut 1 faces at (135.2333, 1.3333, 88.965) along direction (0, 0, -1) blind 1 on bodies 2 bodies 2
chamfer "Chamfer30" distance 3 angle 45 1 edges at (135.15, 2, 87.965) on bodies 2
extrude "Extrude55" cut 1 faces at (135.2333, 15.6667, 30.855) along direction (0, 0, 1) blind 1 on bodies 2 bodies 2
chamfer "Chamfer31" distance 3 angle 45 1 edges at (135.15, 15, 31.855) on bodies 2
extrude "Extrude56" cut 1 faces at (135.2333, 15.6667, 63.91) along direction (0, 0, 1) blind 1 on bodies 2 bodies 2
chamfer "Chamfer32" distance 3 angle 45 1 edges at (135.15, 15, 64.91) on bodies 2
extrude "Extrude57" cut 1 faces at (135.2333, 15.6667, 96.965) along direction (0, 0, 1) blind 1 on bodies 2 bodies 2
chamfer "Chamfer33" distance 3 angle 45 1 edges at (135.15, 15, 97.965) on bodies 2
extrude "Extrude58" cut 1 faces at (135.2333, 15.6667, 88.965) along direction (0, 0, -1) blind 1 on bodies 2 bodies 2
chamfer "Chamfer34" distance 3 angle 45 1 edges at (135.15, 15, 87.965) on bodies 2
extrude "Extrude59" cut 1 faces at (135.2333, 15.6667, 55.91) along direction (0, 0, -1) blind 1 on bodies 2 bodies 2
chamfer "Chamfer35" distance 3 angle 45 1 edges at (135.15, 15, 54.91) on bodies 2
extrude "Extrude60" cut 1 faces at (135.2333, 15.6667, 22.855) along direction (0, 0, -1) blind 1 on bodies 2 bodies 2
chamfer "Chamfer36" distance 3 angle 45 1 edges at (135.15, 15, 21.855) on bodies 2
extrude "Extrude61" cut 1 faces at (36.7, 17, 77.7133) along direction (0, 1, 0) blind 0.25 on bodies 2 bodies 2
extrude "Extrude62" add 1 faces at (93.7667, 18, 58.2433) along direction (0, 1, 0) blind 0.25 on bodies 2 bodies 2
extrude "Extrude63" cut 1 faces at (36.7, 0, 42.1067) along direction (0, -1, 0) blind 0.25 on bodies 2 bodies 2
extrude "Extrude64" add 1 faces at (93.7667, -1, 61.5767) along direction (0, -1, 0) blind 0.25 on bodies 2 bodies 2
extrude "Extrude65" cut 1 faces at (36.7, 11.4167, -0.2) along direction (0, 0, -1) blind 0.25 on bodies 2 bodies 2
extrude "Extrude66" cut 1 faces at (73.4, 5.5833, 120.02) along direction (0, 0, 1) blind 0.25 on bodies 2 bodies 2
extrude "Extrude67" cut 1 faces at (110.1, 5.5833, 1.8667) along direction (1, 0, 0) blind 0.25 on bodies 2 bodies 2
extrude "Extrude68" cut 1 faces at (118.2, 5.5833, 6.5) along direction (0, 0, -1) blind 0.25 on bodies 2 bodies 2
extrude "Extrude69" cut 1 faces at (118.0333, 11.4167, 113.32) along direction (0, 0, 1) blind 0.25 on bodies 2 bodies 2
extrude "Extrude70" add 6 faces at (134.4, 0.6667, 92.2981) (134.4, 0.6667, 59.2431) (134.4, 0.6667, 26.1879) (134.4, 16.3333, 27.5217) (134.4, 16.3333, 60.5769) (134.4, 16.3333, 92.2983) along direction (1, 0, 0) blind 1 on bodies 2 bodies 2
extrude "Extrude71" add 6 faces at (135.4, 17.1667, 92.2983) (135.4, -0.1667, 92.2981) (135.4, -0.1667, 59.2431) (135.4, 17.1667, 60.5769) (135.4, 17.1667, 26.1883) (135.4, -0.1667, 27.5217) along direction (1, 0, 0) blind 0.5 on bodies 2 bodies 2
sketch "Sketch16" plane through (0, 17.25, 0) normal (0, -1, 0) x (1, 0, 0)
  line L0 (0, 120.27) -> (0, -0.45)
  line L1 (0, -0.45) -> (110.35, -0.45)
  line L2 (110.35, -0.45) -> (110.35, 6.25)
  line L3 (110.35, 6.25) -> (133.9, 6.25)
  line L4 (133.9, 6.25) -> (133.9, 113.57)
  line L5 (133.9, 113.57) -> (110.1, 113.57)
  line L6 (110.1, 113.57) -> (110.1, 120.27)
  line L7 (110.1, 120.27) -> (0, 120.27)
  line L8 (110.1, 113.57) -> (-2.7697, 113.57)
  line L9 (-2.7697, 113.57) -> (-2.7697, 6.25)
  line L10 (-2.7697, 6.25) -> (110.1, 6.25)
  line L11 (110.1, 6.25) -> (110.1, 113.57)
  constraint horizontal L8
  constraint vertical L9
  constraint horizontal L10
  constraint vertical L11
  constraint coincident L5.end L6.start
extrude "Extrude72" cut sketch "Sketch16" against normal blind 5 contours L0 L8 L10 L11 bodies 2
sketch "Sketch17" plane through (0, -0.25, 0) normal (0, 1, 0) x (-1, 0, 0)
  line L0 (0, -0.45) -> (0, 120.27)
  line L1 (0, 120.27) -> (-110.1, 120.27)
  line L2 (-110.1, 120.27) -> (-110.1, 113.57)
  line L3 (-110.1, 113.57) -> (-133.9, 113.57)
  line L4 (-133.9, 113.57) -> (-133.9, 6.25)
  line L5 (-133.9, 6.25) -> (-110.35, 6.25)
  line L6 (-110.35, 6.25) -> (-110.35, -0.45)
  line L7 (-110.35, -0.45) -> (0, -0.45)
  line L8 (0, 113.57) -> (-110.35, 113.57)
  line L9 (-110.35, 113.57) -> (-110.35, 6.25)
  line L10 (-110.35, 6.25) -> (0, 6.25)
  line L11 (0, 6.25) -> (0, 113.57)
  point P0 (0, 113.57)
  constraint horizontal L8
  constraint vertical L9
  constraint horizontal L10
  constraint vertical L11
  constraint coincident L5.end L6.start
  constraint coincident P0 L8.start
extrude "Extrude73" cut sketch "Sketch17" against normal blind 10 contours L0 L3 L8 L9 L10 L11 bodies 2
sketch "Sketch18" plane through (0, 18.25, 0) normal (0, 1, 0) x (-1, 0, 0)
  line L0 (0, 6.25) -> (-110.1, 6.25)
  line L1 (-110.1, 6.25) -> (-110.1, 113.57)
  line L2 (-110.1, 113.57) -> (0, 113.57)
  line L3 (0, 113.57) -> (0, 122.02)
  line L4 (0, 122.02) -> (-26.975, 122.02)
  line L5 (-26.975, 122.02) -> (-26.975, 121.52)
  line L6 (-26.975, 121.52) -> (-36.975, 121.52)
  line L7 (-36.975, 121.52) -> (-36.975, 122.02)
  line L8 (-36.975, 122.02) -> (-62.95, 122.02)
  line L9 (-62.95, 122.02) -> (-62.95, 121.52)
  line L10 (-62.95, 121.52) -> (-72.95, 121.52)
  line L11 (-72.95, 121.52) -> (-72.95, 122.02)
  line L12 (-72.95, 122.02) -> (-98.925, 122.02)
  line L13 (-98.925, 122.02) -> (-98.925, 121.52)
  line L14 (-98.925, 121.52) -> (-108.925, 121.52)
  line L15 (-108.925, 121.52) -> (-108.925, 122.02)
  line L16 (-108.925, 122.02) -> (-135.9, 122.02)
  line L17 (-135.9, 122.02) -> (-135.9, -2.2)
  line L18 (-135.9, -2.2) -> (-108.925, -2.2)
  line L19 (-108.925, -2.2) -> (-108.925, -1.7)
  line L20 (-108.925, -1.7) -> (-98.925, -1.7)
  line L21 (-98.925, -1.7) -> (-98.925, -2.2)
  line L22 (-98.925, -2.2) -> (-72.95, -2.2)
  line L23 (-72.95, -2.2) -> (-72.95, -1.7)
  line L24 (-72.95, -1.7) -> (-63.95, -1.7)
  line L25 (-63.95, -1.7) -> (-63.95, -2.2)
  line L26 (-63.95, -2.2) -> (-36.975, -2.2)
  line L27 (-36.975, -2.2) -> (-36.975, -1.7)
  line L28 (-36.975, -1.7) -> (-26.975, -1.7)
  line L29 (-26.975, -1.7) -> (-26.975, -2.2)
  line L30 (-26.975, -2.2) -> (0, -2.2)
  line L31 (0, -2.2) -> (0, 6.25)
  line L32 (0, 6.25) -> (-5, 6.25)
  line L33 (-5, 6.25) -> (-5, 113.57)
  line L34 (-5, 113.57) -> (0, 113.57)
  line L35 (0, 113.57) -> (0, 6.25)
  dimension "d261" = 5
  constraint horizontal L32
  constraint vertical L33
  constraint horizontal L34
  constraint vertical L35
  constraint coincident L0.start L31.end
  measures "d261" distance of L0.start L32.end
extrude "Extrude74" add sketch "Sketch18" against normal blind 1 contours L0 L2 L32 L33 L34 L35 bodies 2
chamfer "Chamfer37" distance 25 angle 65 2 edges at (5, 17.75, 6.25) (5, 17.75, 113.57) measured on face at (40.0333, 17.9167, 6.25) measured on face at (75.0667, 17.5833, 113.57) on bodies 2
sketch "Sketch19" plane through (0, -1.25, 0) normal (0, -1, 0) x (1, 0, 0)
  line L0 (0, 113.57) -> (110.35, 113.57)
  line L1 (110.35, 113.57) -> (110.35, 6.25)
  line L2 (110.35, 6.25) -> (0, 6.25)
  line L3 (0, 6.25) -> (0, -2.2)
  line L4 (0, -2.2) -> (27.975, -2.2)
  line L5 (27.975, -2.2) -> (27.975, -1.7)
  line L6 (27.975, -1.7) -> (36.975, -1.7)
  line L7 (36.975, -1.7) -> (36.975, -2.2)
  line L8 (36.975, -2.2) -> (62.95, -2.2)
  line L9 (62.95, -2.2) -> (62.95, -1.7)
  line L10 (62.95, -1.7) -> (72.95, -1.7)
  line L11 (72.95, -1.7) -> (72.95, -2.2)
  line L12 (72.95, -2.2) -> (98.925, -2.2)
  line L13 (98.925, -2.2) -> (98.925, -1.7)
  line L14 (98.925, -1.7) -> (108.925, -1.7)
  line L15 (108.925, -1.7) -> (108.925, -2.2)
  line L16 (108.925, -2.2) -> (135.9, -2.2)
  line L17 (135.9, -2.2) -> (135.9, 122.02)
  line L18 (135.9, 122.02) -> (108.925, 122.02)
  line L19 (108.925, 122.02) -> (108.925, 121.52)
  line L20 (108.925, 121.52) -> (98.925, 121.52)
  line L21 (98.925, 121.52) -> (98.925, 122.02)
  line L22 (98.925, 122.02) -> (72.95, 122.02)
  line L23 (72.95, 122.02) -> (72.95, 121.52)
  line L24 (72.95, 121.52) -> (62.95, 121.52)
  line L25 (62.95, 121.52) -> (62.95, 122.02)
  line L26 (62.95, 122.02) -> (36.975, 122.02)
  line L27 (36.975, 122.02) -> (36.975, 121.52)
  line L28 (36.975, 121.52) -> (26.975, 121.52)
  line L29 (26.975, 121.52) -> (26.975, 122.02)
  line L30 (26.975, 122.02) -> (0, 122.02)
  line L31 (0, 122.02) -> (0, 113.57)
  line L32 (0, 6.25) -> (5, 6.25)
  line L33 (5, 6.25) -> (5, 113.57)
  line L34 (5, 113.57) -> (0, 113.57)
  line L35 (0, 113.57) -> (0, 6.25)
  dimension "d266" = 5
  constraint horizontal L32
  constraint vertical L33
  constraint horizontal L34
  constraint vertical L35
  constraint coincident L2.end L3.start
  measures "d266" distance of L2.end L32.end
extrude "Extrude75" add sketch "Sketch19" along normal blind 1 separate body contours L0 L2 L32 L33 L34 L35 makes body 3
extrude "Extrude76" add 1 faces at (3.3333, -1.25, 42.0233) along direction (0, 1, 0) blind 1 on bodies 3 bodies 3 2
extrude "Extrude77" cut 1 faces at (3.3333, -2.25, 42.0233) along direction (0, 1, 0) blind 1 on bodies 3 bodies 3